Autodesk Fusion 360 part; units mm, degrees
(part 6 of 18)
  arc A594 (213.8474, -42.2017) -> (215.0474, -42.2017) centre (214.4474, -42.2017) ccw
  arc A595 (215.0474, -42.2017) -> (213.8474, -42.2017) centre (214.4474, -42.2017) ccw
  arc A596 (210.3474, -44.4557) -> (211.5474, -44.4557) centre (210.9474, -44.4557) ccw
  arc A597 (211.5474, -44.4557) -> (210.3474, -44.4557) centre (210.9474, -44.4557) ccw
  arc A598 (215.0474, -23.1516) -> (213.8474, -23.1516) centre (214.4474, -23.1516) ccw
  arc A599 (213.8474, -23.1516) -> (215.0474, -23.1516) centre (214.4474, -23.1516) ccw
  arc A600 (211.5474, -25.4057) -> (210.3474, -25.4057) centre (210.9474, -25.4057) ccw
  arc A601 (210.3474, -25.4057) -> (211.5474, -25.4057) centre (210.9474, -25.4057) ccw
  arc A602 (213.8474, -80.3272) -> (215.0474, -80.3272) centre (214.4474, -80.3272) ccw
  arc A603 (215.0474, -80.3272) -> (213.8474, -80.3272) centre (214.4474, -80.3272) ccw
  arc A604 (210.3474, -82.5812) -> (211.5474, -82.5812) centre (210.9474, -82.5812) ccw
  arc A605 (211.5474, -82.5812) -> (210.3474, -82.5812) centre (210.9474, -82.5812) ccw
  arc A606 (195.9974, -42.2017) -> (194.7974, -42.2017) centre (195.3974, -42.2017) ccw
  arc A607 (194.7974, -42.2017) -> (195.9974, -42.2017) centre (195.3974, -42.2017) ccw
  arc A608 (192.4974, -44.4557) -> (191.2974, -44.4557) centre (191.8974, -44.4557) ccw
  arc A609 (191.2974, -44.4557) -> (192.4974, -44.4557) centre (191.8974, -44.4557) ccw
  arc A610 (175.1224, -4.318) -> (176.9224, -4.318) centre (176.0224, -4.318) ccw
  arc A611 (176.9224, -4.318) -> (175.1224, -4.318) centre (176.0224, -4.318) ccw
  line L3563 (172.5823, -3.418) -> (174.3823, -3.418)
  line L3564 (174.3823, -5.218) -> (172.5823, -5.218)
  line L3565 (172.5823, -5.218) -> (172.5823, -3.418)
  line L3566 (174.3823, -3.418) -> (174.3823, -5.218)
  line L3567 (184.8974, -50.5184) -> (198.8974, -50.5184)
  line L3568 (198.8974, -50.5184) -> (198.8974, -64.5184)
  line L3569 (184.8974, -64.5184) -> (184.8974, -50.5184)
  line L3570 (198.8974, -64.5184) -> (184.8974, -64.5184)
  line L3571 (179.8474, -69.5811) -> (179.8474, -83.5812)
  line L3572 (165.8473, -83.5812) -> (165.8473, -69.5811)
  line L3573 (165.8473, -69.5811) -> (179.8474, -69.5811)
  line L3574 (179.8474, -83.5812) -> (165.8473, -83.5812)
  line L3575 (165.8473, -50.5184) -> (179.8474, -50.5184)
  line L3576 (165.8473, -64.5184) -> (165.8473, -50.5184)
  line L3577 (179.8474, -50.5184) -> (179.8474, -64.5184)
  line L3578 (179.8474, -64.5184) -> (165.8473, -64.5184)
  line L3579 (179.8474, -45.4557) -> (165.8473, -45.4557)
  line L3580 (179.8474, -31.4557) -> (179.8474, -45.4557)
  line L3581 (165.8473, -45.4557) -> (165.8473, -31.4557)
  line L3582 (165.8473, -31.4557) -> (179.8474, -31.4557)
  line L3583 (179.8474, -26.4057) -> (165.8473, -26.4057)
  line L3584 (179.8474, -12.4056) -> (179.8474, -26.4057)
  line L3585 (165.8473, -26.4057) -> (165.8473, -12.4056)
  line L3586 (165.8473, -12.4056) -> (179.8474, -12.4056)
  line L3587 (160.7973, -83.5812) -> (146.7973, -83.5812)
  line L3588 (146.7973, -69.5811) -> (160.7973, -69.5811)
  line L3589 (160.7973, -69.5811) -> (160.7973, -83.5812)
  line L3590 (146.7973, -83.5812) -> (146.7973, -69.5811)
  line L3591 (160.7973, -45.4557) -> (146.7973, -45.4557)
  line L3592 (146.7973, -45.4557) -> (146.7973, -31.4557)
  line L3593 (160.7973, -31.4557) -> (160.7973, -45.4557)
  line L3594 (146.7973, -31.4557) -> (160.7973, -31.4557)
  line L3595 (160.7973, -50.5184) -> (160.7973, -64.5184)
  line L3596 (160.7973, -64.5184) -> (146.7973, -64.5184)
  line L3597 (146.7973, -64.5184) -> (146.7973, -50.5184)
  line L3598 (146.7973, -50.5184) -> (160.7973, -50.5184)
  line L3599 (160.7973, -12.4056) -> (160.7973, -26.4057)
  line L3600 (146.7973, -12.4056) -> (160.7973, -12.4056)
  line L3601 (146.7973, -26.4057) -> (146.7973, -12.4056)
  line L3602 (160.7973, -26.4057) -> (146.7973, -26.4057)
  line L3603 (141.7473, -64.5184) -> (127.7473, -64.5184)
  line L3604 (141.7473, -50.5184) -> (141.7473, -64.5184)
  line L3605 (127.7473, -50.5184) -> (141.7473, -50.5184)
  line L3606 (127.7473, -64.5184) -> (127.7473, -50.5184)
  line L3607 (141.7473, -45.4557) -> (127.7473, -45.4557)
  line L3608 (127.7473, -45.4557) -> (127.7473, -31.4557)
  line L3609 (141.7473, -31.4557) -> (141.7473, -45.4557)
  line L3610 (127.7473, -31.4557) -> (141.7473, -31.4557)
  line L3611 (127.7473, -12.4056) -> (141.7473, -12.4056)
  line L3612 (141.7473, -12.4056) -> (141.7473, -26.4057)
  line L3613 (141.7473, -26.4057) -> (127.7473, -26.4057)
  line L3614 (127.7473, -26.4057) -> (127.7473, -12.4056)
  line L3615 (141.7473, -83.5812) -> (127.7473, -83.5812)
  line L3616 (127.7473, -83.5812) -> (127.7473, -69.5811)
  line L3617 (127.7473, -69.5811) -> (141.7473, -69.5811)
  line L3618 (141.7473, -69.5811) -> (141.7473, -83.5812)
  line L3619 (108.6972, -69.5811) -> (122.6972, -69.5811)
  line L3620 (122.6972, -83.5812) -> (108.6972, -83.5812)
  line L3621 (108.6972, -83.5812) -> (108.6972, -69.5811)
  line L3622 (122.6972, -69.5811) -> (122.6972, -83.5812)
  line L3623 (108.6972, -64.5184) -> (108.6972, -50.5184)
  line L3624 (122.6972, -64.5184) -> (108.6972, -64.5184)
  line L3625 (122.6972, -50.5184) -> (122.6972, -64.5184)
  line L3626 (108.6972, -50.5184) -> (122.6972, -50.5184)
  line L3627 (108.6972, -12.4056) -> (122.6972, -12.4056)
  line L3628 (108.6972, -26.4057) -> (108.6972, -12.4056)
  line L3629 (122.6972, -26.4057) -> (108.6972, -26.4057)
  line L3630 (122.6972, -12.4056) -> (122.6972, -26.4057)
  line L3631 (122.6972, -45.4557) -> (108.6972, -45.4557)
  line L3632 (122.6972, -31.4557) -> (122.6972, -45.4557)
  line L3633 (108.6972, -31.4557) -> (122.6972, -31.4557)
  line L3634 (108.6972, -45.4557) -> (108.6972, -31.4557)
  line L3635 (89.6472, -26.4057) -> (89.6472, -12.4056)
  line L3636 (103.6472, -12.4056) -> (103.6472, -26.4057)
  line L3637 (103.6472, -26.4057) -> (89.6472, -26.4057)
  line L3638 (89.6472, -12.4056) -> (103.6472, -12.4056)
  line L3639 (89.6472, -31.4557) -> (103.6472, -31.4557)
  line L3640 (89.6472, -45.4557) -> (89.6472, -31.4557)
  line L3641 (103.6472, -31.4557) -> (103.6472, -45.4557)
  line L3642 (103.6472, -45.4557) -> (89.6472, -45.4557)
  line L3643 (89.6472, -83.5812) -> (89.6472, -69.5811)
  line L3644 (103.6472, -83.5812) -> (89.6472, -83.5812)
  line L3645 (89.6472, -69.5811) -> (103.6472, -69.5811)
  line L3646 (103.6472, -69.5811) -> (103.6472, -83.5812)
  line L3647 (103.6472, -64.5184) -> (89.6472, -64.5184)
  line L3648 (89.6472, -50.5184) -> (103.6472, -50.5184)
  line L3649 (103.6472, -50.5184) -> (103.6472, -64.5184)
  line L3650 (89.6472, -64.5184) -> (89.6472, -50.5184)
  line L3651 (198.8974, -69.5811) -> (198.8974, -83.5812)
  line L3652 (184.8974, -83.5812) -> (184.8974, -69.5811)
  line L3653 (184.8974, -69.5811) -> (198.8974, -69.5811)
  line L3654 (198.8974, -83.5812) -> (184.8974, -83.5812)
  line L3655 (198.8974, -26.4057) -> (184.8974, -26.4057)
  line L3656 (184.8974, -12.4056) -> (198.8974, -12.4056)
  line L3657 (198.8974, -12.4056) -> (198.8974, -26.4057)
  line L3658 (184.8974, -26.4057) -> (184.8974, -12.4056)
  line L3659 (84.5972, -83.5812) -> (70.5971, -83.5812)
  line L3660 (70.5971, -69.5811) -> (84.5972, -69.5811)
  line L3661 (84.5972, -69.5811) -> (84.5972, -83.5812)
  line L3662 (70.5971, -83.5812) -> (70.5971, -69.5811)
  line L3663 (84.5972, -45.4557) -> (70.5971, -45.4557)
  line L3664 (84.5972, -31.4557) -> (84.5972, -45.4557)
  line L3665 (70.5971, -31.4557) -> (84.5972, -31.4557)
  line L3666 (70.5971, -45.4557) -> (70.5971, -31.4557)
  line L3667 (84.5972, -12.4056) -> (84.5972, -26.4057)
  line L3668 (84.5972, -26.4057) -> (70.5971, -26.4057)
  line L3669 (70.5971, -26.4057) -> (70.5971, -12.4056)
  line L3670 (70.5971, -12.4056) -> (84.5972, -12.4056)
  line L3671 (70.5971, -64.5184) -> (70.5971, -50.5184)
  line L3672 (84.5972, -64.5184) -> (70.5971, -64.5184)
  line L3673 (70.5971, -50.5184) -> (84.5972, -50.5184)
  line L3674 (84.5972, -50.5184) -> (84.5972, -64.5184)
  line L3675 (65.5471, -83.5812) -> (51.5471, -83.5812)
  line L3676 (51.5471, -69.5811) -> (65.5471, -69.5811)
  line L3677 (65.5471, -69.5811) -> (65.5471, -83.5812)
  line L3678 (51.5471, -83.5812) -> (51.5471, -69.5811)
  line L3679 (51.5471, -50.5184) -> (65.5471, -50.5184)
  line L3680 (65.5471, -64.5184) -> (51.5471, -64.5184)
  line L3681 (65.5471, -50.5184) -> (65.5471, -64.5184)
  line L3682 (51.5471, -64.5184) -> (51.5471, -50.5184)
  line L3683 (51.5471, -31.4557) -> (65.5471, -31.4557)
  line L3684 (65.5471, -45.4557) -> (51.5471, -45.4557)
  line L3685 (51.5471, -45.4557) -> (51.5471, -31.4557)
  line L3686 (65.5471, -31.4557) -> (65.5471, -45.4557)
  line L3687 (32.4971, -64.5184) -> (32.4971, -50.5184)
  line L3688 (32.4971, -50.5184) -> (46.4971, -50.5184)
  line L3689 (46.4971, -50.5184) -> (46.4971, -64.5184)
  line L3690 (46.4971, -64.5184) -> (32.4971, -64.5184)
  line L3691 (32.4971, -83.5812) -> (32.4971, -69.5811)
  line L3692 (46.4971, -69.5811) -> (46.4971, -83.5812)
  line L3693 (32.4971, -69.5811) -> (46.4971, -69.5811)
  line L3694 (46.4971, -83.5812) -> (32.4971, -83.5812)
  line L3695 (13.447, -83.5812) -> (13.447, -69.5811)
  line L3696 (13.447, -69.5811) -> (27.4471, -69.5811)
  line L3697 (27.4471, -83.5812) -> (13.447, -83.5812)
  line L3698 (27.4471, -69.5811) -> (27.4471, -83.5812)
  line L3699 (-5.603, -83.5812) -> (-5.603, -69.5811)
  line L3700 (8.397, -83.5812) -> (-5.603, -83.5812)
  line L3701 (8.397, -69.5811) -> (8.397, -83.5812)
  line L3702 (-5.603, -69.5811) -> (8.397, -69.5811)
  line L3703 (65.5471, -12.4056) -> (65.5471, -26.4057)
  line L3704 (65.5471, -26.4057) -> (51.5471, -26.4057)
  line L3705 (51.5471, -12.4056) -> (65.5471, -12.4056)
  line L3706 (51.5471, -26.4057) -> (51.5471, -12.4056)
  line L3707 (46.4971, -31.4557) -> (46.4971, -45.4557)
  line L3708 (46.4971, -45.4557) -> (32.4971, -45.4557)
  line L3709 (32.4971, -31.4557) -> (46.4971, -31.4557)
  line L3710 (32.4971, -45.4557) -> (32.4971, -31.4557)
  line L3711 (46.4971, -26.4057) -> (32.4971, -26.4057)
  line L3712 (32.4971, -12.4056) -> (46.4971, -12.4056)
  line L3713 (46.4971, -12.4056) -> (46.4971, -26.4057)
  line L3714 (32.4971, -26.4057) -> (32.4971, -12.4056)
  line L3715 (13.447, -26.4057) -> (13.447, -12.4056)
  line L3716 (13.447, -12.4056) -> (27.4471, -12.4056)
  line L3717 (27.4471, -26.4057) -> (13.447, -26.4057)
  line L3718 (27.4471, -12.4056) -> (27.4471, -26.4057)
  line L3719 (13.447, -64.5184) -> (13.447, -50.5184)
  line L3720 (27.4471, -50.5184) -> (27.4471, -64.5184)
  line L3721 (13.447, -50.5184) -> (27.4471, -50.5184)
  line L3722 (27.4471, -64.5184) -> (13.447, -64.5184)
  line L3723 (13.447, -31.4557) -> (27.4471, -31.4557)
  line L3724 (27.4471, -31.4557) -> (27.4471, -45.4557)
  line L3725 (13.447, -45.4557) -> (13.447, -31.4557)
  line L3726 (27.4471, -45.4557) -> (13.447, -45.4557)
  line L3727 (-5.603, -12.4056) -> (8.397, -12.4056)
  line L3728 (-5.603, -26.4057) -> (-5.603, -12.4056)
  line L3729 (8.397, -12.4056) -> (8.397, -26.4057)
  line L3730 (8.397, -26.4057) -> (-5.603, -26.4057)
  line L3731 (-5.603, -45.4557) -> (-5.603, -31.4557)
  line L3732 (8.397, -31.4557) -> (8.397, -45.4557)
  line L3733 (-5.603, -31.4557) -> (8.397, -31.4557)
  line L3734 (8.397, -45.4557) -> (-5.603, -45.4557)
  line L3735 (-5.603, -50.5184) -> (8.397, -50.5184)
  line L3736 (-5.603, -64.5184) -> (-5.603, -50.5184)
  line L3737 (8.397, -50.5184) -> (8.397, -64.5184)
  line L3738 (8.397, -64.5184) -> (-5.603, -64.5184)
  line L3739 (203.9474, -64.5184) -> (203.9474, -50.5184)
  line L3740 (217.9474, -64.5184) -> (203.9474, -64.5184)
  line L3741 (217.9474, -50.5184) -> (217.9474, -64.5184)
  line L3742 (203.9474, -50.5184) -> (217.9474, -50.5184)
  line L3743 (203.9474, -45.4557) -> (203.9474, -31.4557)
  line L3744 (203.9474, -31.4557) -> (217.9474, -31.4557)
  line L3745 (217.9474, -31.4557) -> (217.9474, -45.4557)
  line L3746 (217.9474, -45.4557) -> (203.9474, -45.4557)
  line L3747 (203.9474, -12.4056) -> (217.9474, -12.4056)
  line L3748 (217.9474, -12.4056) -> (217.9474, -26.4057)
  line L3749 (203.9474, -26.4057) -> (203.9474, -12.4056)
  line L3750 (217.9474, -26.4057) -> (203.9474, -26.4057)
  line L3751 (203.9474, -69.5811) -> (217.9474, -69.5811)
  line L3752 (217.9474, -83.5812) -> (203.9474, -83.5812)
  line L3753 (217.9474, -69.5811) -> (217.9474, -83.5812)
  line L3754 (203.9474, -83.5812) -> (203.9474, -69.5811)
  line L3755 (184.8974, -45.4557) -> (184.8974, -31.4557)
  line L3756 (184.8974, -31.4557) -> (198.8974, -31.4557)
  line L3757 (198.8974, -31.4557) -> (198.8974, -45.4557)
  line L3758 (198.8974, -45.4557) -> (184.8974, -45.4557)
  arc A612 (206.9597, -6.1629) -> (207.1096, -6.1629) centre (207.0347, -6.1629) ccw
  arc A613 (207.1096, -6.1629) -> (206.9597, -6.1629) centre (207.0347, -6.1629) ccw
  arc A614 (212.2667, -3.8099) -> (212.0665, -3.8099) centre (212.1666, -3.8099) ccw
  arc A615 (212.0665, -3.8099) -> (212.2667, -3.8099) centre (212.1666, -3.8099) ccw
  arc A616 (-2.1624, -5.4611) -> (6.4883, -5.4611) centre (2.1629, -5.4611) ccw
  arc A617 (6.4883, -5.4611) -> (-2.1624, -5.4611) centre (2.1629, -5.4611) ccw
  arc A618 (5.5157, -5.4611) -> (-1.1899, -5.4611) centre (2.1629, -5.4611) ccw
  arc A619 (-1.1899, -5.4611) -> (5.5157, -5.4611) centre (2.1629, -5.4611) ccw
  arc A620 (5.2109, -5.4611) -> (-0.8851, -5.4611) centre (2.1629, -5.4611) ccw
  arc A621 (-0.8851, -5.4611) -> (5.2109, -5.4611) centre (2.1629, -5.4611) ccw
  line L3759 (181.2044, -1.3566) -> (181.2044, -3.0235)
  line L3760 (181.2044, 2.4608) -> (181.2044, 0.9765)
  line L3761 (190.1444, -1.3566) -> (190.1444, -3.0235)
  line L3762 (190.1444, 2.411) -> (190.1444, 0.9765)
  line L3763 (181.2044, 2.4608) -> (190.1444, 2.411)
  line L3764 (200.2342, -1.2444) -> (199.2753, -1.2444)
  line L3765 (199.2753, -1.2444) -> (199.2753, -2.5656)
  line L3766 (199.2753, -2.5656) -> (200.2342, -2.5656)
  line L3767 (201.0866, -1.2444) -> (202.0455, -1.2444)
  line L3768 (202.0455, -1.2444) -> (202.0455, -2.5656)
  line L3769 (202.0455, -2.5656) -> (201.0866, -2.5656)
  line L3770 (213.977, -5.1867) -> (214.6507, -5.1867)
  line L3771 (214.6507, -5.1867) -> (214.6507, -5.8604)
  line L3772 (213.977, -12.3392) -> (214.6507, -12.3392)
  line L3773 (214.6507, -12.3392) -> (214.6507, -11.6655)
  line L3774 (208.172, -5.1867) -> (207.4983, -5.1867)
  line L3775 (207.4983, -5.1867) -> (207.4983, -5.8604)
  line L3776 (208.172, -12.3392) -> (207.4983, -12.3392)
  line L3777 (207.4983, -12.3392) -> (207.4983, -11.6655)
  line L3778 (188.1326, -7.3916) -> (189.0915, -7.3916)
  line L3779 (189.0915, -7.3916) -> (189.0915, -6.0704)
  line L3780 (189.0915, -6.0704) -> (188.1326, -6.0704)
  line L3781 (187.2802, -7.3916) -> (186.3213, -7.3916)
  line L3782 (186.3213, -7.3916) -> (186.3213, -6.0704)
  line L3783 (186.3213, -6.0704) -> (187.2802, -6.0704)
  line L3784 (182.7082, -6.0704) -> (181.7493, -6.0704)
  line L3785 (181.7493, -6.0704) -> (181.7493, -7.3916)
  line L3786 (181.7493, -7.3916) -> (182.7082, -7.3916)
  line L3787 (183.5606, -6.0704) -> (184.5195, -6.0704)
  line L3788 (184.5195, -6.0704) -> (184.5195, -7.3916)
  line L3789 (184.5195, -7.3916) -> (183.5606, -7.3916)
  line L3790 (208.6489, -3.8645) -> (208.6489, -0.7644)
  line L3791 (211.749, -0.7644) -> (208.6489, -0.7644)
  line L3792 (211.7477, -3.8645) -> (211.7477, -0.7644)
  line L3793 (208.6489, -3.8886) -> (209.4871, -3.8886)
  line L3794 (210.9095, -3.8886) -> (211.7477, -3.8886)
  arc A622 (209.5125, -3.8886) -> (210.9095, -3.8886) centre (210.211, -4.1061) cw
  line L3795 (141.7615, -77.4607) -> (141.7615, -77.7869)
  line L3796 (141.7615, -75.9344) -> (141.7615, -76.2604)
  line L3797 (138.9091, -75.9344) -> (141.7615, -75.9344)
  line L3798 (138.9091, -77.7869) -> (141.7615, -77.7869)
  line L3799 (139.3639, -77.7867) -> (139.3639, -75.9343)
  line L3800 (138.6805, -77.3568) -> (138.6805, -77.863)
  line L3801 (138.9853, -77.3568) -> (138.6805, -77.3568)
  line L3802 (138.6805, -77.863) -> (138.9853, -77.863)
  line L3803 (138.9853, -77.863) -> (138.9853, -77.3568)
  line L3804 (138.6805, -76.3644) -> (138.6805, -75.8582)
  line L3805 (138.9853, -75.8582) -> (138.9853, -76.3644)
  line L3806 (138.9853, -76.3644) -> (138.6805, -76.3644)
  line L3807 (138.6805, -75.8582) -> (138.9853, -75.8582)
  line L3808 (141.7615, -20.2852) -> (141.7615, -20.6114)
  line L3809 (141.7615, -18.7589) -> (141.7615, -19.0849)
  line L3810 (138.9091, -18.7589) -> (141.7615, -18.7589)
  line L3811 (138.9091, -20.6114) -> (141.7615, -20.6114)
  line L3812 (139.3639, -20.6112) -> (139.3639, -18.7588)
  line L3813 (138.6805, -20.6874) -> (138.9853, -20.6874)
  line L3814 (138.6805, -20.1812) -> (138.6805, -20.6874)
  line L3815 (138.9853, -20.6874) -> (138.9853, -20.1812)
  line L3816 (138.9853, -20.1812) -> (138.6805, -20.1812)
  line L3817 (138.9853, -19.1888) -> (138.6805, -19.1888)
  line L3818 (138.6805, -19.1888) -> (138.6805, -18.6826)
  line L3819 (138.9853, -18.6826) -> (138.9853, -19.1888)
  line L3820 (138.6805, -18.6826) -> (138.9853, -18.6826)
  line L3821 (141.7615, -39.3352) -> (141.7615, -39.6614)
  line L3822 (141.7615, -37.8089) -> (141.7615, -38.135)
  line L3823 (138.9091, -37.8089) -> (141.7615, -37.8089)
  line L3824 (138.9091, -39.6614) -> (141.7615, -39.6614)
  line L3825 (139.3639, -39.6613) -> (139.3639, -37.8089)
  line L3826 (138.9853, -39.7375) -> (138.9853, -39.2313)
  line L3827 (138.6805, -39.7375) -> (138.9853, -39.7375)
  line L3828 (138.9853, -39.2313) -> (138.6805, -39.2313)
  line L3829 (138.6805, -39.2313) -> (138.6805, -39.7375)
  line L3830 (138.6805, -37.7327) -> (138.9853, -37.7327)
  line L3831 (138.9853, -38.2389) -> (138.6805, -38.2389)
  line L3832 (138.6805, -38.2389) -> (138.6805, -37.7327)
  line L3833 (138.9853, -37.7327) -> (138.9853, -38.2389)
  line L3834 (141.7615, -58.3979) -> (141.7615, -58.7242)
  line L3835 (141.7615, -56.8716) -> (141.7615, -57.1977)
  line L3836 (138.9091, -56.8716) -> (141.7615, -56.8716)
  line L3837 (138.9091, -58.7242) -> (141.7615, -58.7242)
  line L3838 (139.3639, -58.724) -> (139.3639, -56.8716)
  line L3839 (138.6805, -58.8002) -> (138.9853, -58.8002)
  line L3840 (138.9853, -58.8002) -> (138.9853, -58.294)
  line L3841 (138.9853, -58.294) -> (138.6805, -58.294)
  line L3842 (138.6805, -58.294) -> (138.6805, -58.8002)
  line L3843 (138.6805, -56.7954) -> (138.9853, -56.7954)
  line L3844 (138.9853, -57.3016) -> (138.6805, -57.3016)
  line L3845 (138.6805, -57.3016) -> (138.6805, -56.7954)
  line L3846 (138.9853, -56.7954) -> (138.9853, -57.3016)
  line L3847 (160.8115, -20.2852) -> (160.8115, -20.6114)
  line L3848 (160.8115, -18.7589) -> (160.8115, -19.0849)
  line L3849 (157.9591, -18.7589) -> (160.8115, -18.7589)
  line L3850 (157.9591, -20.6114) -> (160.8115, -20.6114)
  line L3851 (158.4139, -20.6112) -> (158.4139, -18.7588)
  line L3852 (158.0353, -20.1812) -> (157.7305, -20.1812)
  line L3853 (157.7305, -20.1812) -> (157.7305, -20.6874)
  line L3854 (157.7305, -20.6874) -> (158.0353, -20.6874)
  line L3855 (158.0353, -20.6874) -> (158.0353, -20.1812)
  line L3856 (157.7305, -18.6826) -> (158.0353, -18.6826)
  line L3857 (157.7305, -19.1888) -> (157.7305, -18.6826)
  line L3858 (158.0353, -19.1888) -> (157.7305, -19.1888)
  line L3859 (158.0353, -18.6826) -> (158.0353, -19.1888)
  line L3860 (160.8115, -77.4607) -> (160.8115, -77.7869)
  line L3861 (160.8115, -75.9344) -> (160.8115, -76.2604)
  line L3862 (157.9591, -75.9344) -> (160.8115, -75.9344)
  line L3863 (157.9591, -77.7869) -> (160.8115, -77.7869)
  line L3864 (158.4139, -77.7867) -> (158.4139, -75.9343)
  line L3865 (157.7305, -77.863) -> (158.0353, -77.863)
  line L3866 (158.0353, -77.863) -> (158.0353, -77.3568)
  line L3867 (158.0353, -77.3568) -> (157.7305, -77.3568)
  line L3868 (157.7305, -77.3568) -> (157.7305, -77.863)
  line L3869 (158.0353, -76.3644) -> (157.7305, -76.3644)
  line L3870 (157.7305, -75.8582) -> (158.0353, -75.8582)
  line L3871 (157.7305, -76.3644) -> (157.7305, -75.8582)
  line L3872 (158.0353, -75.8582) -> (158.0353, -76.3644)
  line L3873 (160.8115, -58.3979) -> (160.8115, -58.7242)
  line L3874 (160.8115, -56.8716) -> (160.8115, -57.1977)
  line L3875 (157.9591, -56.8716) -> (160.8115, -56.8716)
  line L3876 (157.9591, -58.7242) -> (160.8115, -58.7242)
  line L3877 (158.4139, -58.724) -> (158.4139, -56.8716)
  line L3878 (158.0353, -58.8002) -> (158.0353, -58.294)
  line L3879 (158.0353, -58.294) -> (157.7305, -58.294)
  line L3880 (157.7305, -58.8002) -> (158.0353, -58.8002)
  line L3881 (157.7305, -58.294) -> (157.7305, -58.8002)
  line L3882 (158.0353, -56.7954) -> (158.0353, -57.3016)
  line L3883 (157.7305, -56.7954) -> (158.0353, -56.7954)
  line L3884 (157.7305, -57.3016) -> (157.7305, -56.7954)
  line L3885 (158.0353, -57.3016) -> (157.7305, -57.3016)
  line L3886 (160.8115, -39.3352) -> (160.8115, -39.6614)
  line L3887 (160.8115, -37.8089) -> (160.8115, -38.135)
  line L3888 (157.9591, -37.8089) -> (160.8115, -37.8089)
  line L3889 (157.9591, -39.6614) -> (160.8115, -39.6614)
  line L3890 (158.4139, -39.6613) -> (158.4139, -37.8089)
  line L3891 (158.0353, -39.2313) -> (157.7305, -39.2313)
  line L3892 (157.7305, -39.2313) -> (157.7305, -39.7375)
  line L3893 (158.0353, -39.7375) -> (158.0353, -39.2313)
  line L3894 (157.7305, -39.7375) -> (158.0353, -39.7375)
  line L3895 (158.0353, -37.7327) -> (158.0353, -38.2389)
  line L3896 (157.7305, -37.7327) -> (158.0353, -37.7327)
  line L3897 (158.0353, -38.2389) -> (157.7305, -38.2389)
  line L3898 (157.7305, -38.2389) -> (157.7305, -37.7327)
  line L3899 (179.8616, -20.2852) -> (179.8616, -20.6114)
  line L3900 (179.8616, -18.7589) -> (179.8616, -19.0849)
  line L3901 (177.0092, -18.7589) -> (179.8616, -18.7589)
  line L3902 (177.0091, -20.6114) -> (179.8616, -20.6114)
  line L3903 (177.464, -20.6112) -> (177.464, -18.7588)
  line L3904 (177.0854, -20.1812) -> (176.7806, -20.1812)
  line L3905 (177.0854, -20.6874) -> (177.0854, -20.1812)
  line L3906 (176.7806, -20.6874) -> (177.0854, -20.6874)
  line L3907 (176.7806, -20.1812) -> (176.7806, -20.6874)
  line L3908 (177.0854, -19.1888) -> (176.7806, -19.1888)
  line L3909 (176.7806, -19.1888) -> (176.7806, -18.6826)
  line L3910 (176.7806, -18.6826) -> (177.0854, -18.6826)
  line L3911 (177.0854, -18.6826) -> (177.0854, -19.1888)
  line L3912 (179.8616, -77.4607) -> (179.8616, -77.7869)
  line L3913 (179.8616, -75.9344) -> (179.8616, -76.2604)
  line L3914 (177.0092, -75.9344) -> (179.8616, -75.9344)
  line L3915 (177.0091, -77.7869) -> (179.8616, -77.7869)
  line L3916 (177.464, -77.7867) -> (177.464, -75.9343)
  line L3917 (176.7806, -77.3568) -> (176.7806, -77.863)
  line L3918 (177.0854, -77.3568) -> (176.7806, -77.3568)
  line L3919 (176.7806, -77.863) -> (177.0854, -77.863)
  line L3920 (177.0854, -77.863) -> (177.0854, -77.3568)
  line L3921 (176.7806, -76.3644) -> (176.7806, -75.8582)
  line L3922 (177.0854, -75.8582) -> (177.0854, -76.3644)
  line L3923 (176.7806, -75.8582) -> (177.0854, -75.8582)
  line L3924 (177.0854, -76.3644) -> (176.7806, -76.3644)
  line L3925 (179.8616, -58.3979) -> (179.8616, -58.7242)
  line L3926 (179.8616, -56.8716) -> (179.8616, -57.1977)
  line L3927 (177.0092, -56.8716) -> (179.8616, -56.8716)
  line L3928 (177.0091, -58.7242) -> (179.8616, -58.7242)
  line L3929 (177.464, -58.724) -> (177.464, -56.8716)
  line L3930 (177.0854, -58.294) -> (176.7806, -58.294)
  line L3931 (176.7806, -58.8002) -> (177.0854, -58.8002)
  line L3932 (177.0854, -58.8002) -> (177.0854, -58.294)
  line L3933 (176.7806, -58.294) -> (176.7806, -58.8002)
  line L3934 (177.0854, -56.7954) -> (177.0854, -57.3016)
  line L3935 (177.0854, -57.3016) -> (176.7806, -57.3016)
  line L3936 (176.7806, -57.3016) -> (176.7806, -56.7954)
  line L3937 (176.7806, -56.7954) -> (177.0854, -56.7954)
  line L3938 (179.8616, -39.3352) -> (179.8616, -39.6614)
  line L3939 (179.8616, -37.8089) -> (179.8616, -38.135)
  line L3940 (177.0092, -37.8089) -> (179.8616, -37.8089)
  line L3941 (177.0091, -39.6614) -> (179.8616, -39.6614)
  line L3942 (177.464, -39.6613) -> (177.464, -37.8089)
  line L3943 (176.7806, -39.7375) -> (177.0854, -39.7375)
  line L3944 (177.0854, -39.7375) -> (177.0854, -39.2313)
  line L3945 (176.7806, -39.2313) -> (176.7806, -39.7375)
  line L3946 (177.0854, -39.2313) -> (176.7806, -39.2313)
  line L3947 (176.7806, -37.7327) -> (177.0854, -37.7327)
  line L3948 (176.7806, -38.2389) -> (176.7806, -37.7327)
  line L3949 (177.0854, -37.7327) -> (177.0854, -38.2389)
  line L3950 (177.0854, -38.2389) -> (176.7806, -38.2389)
  line L3951 (103.6614, -77.4607) -> (103.6614, -77.7869)
  line L3952 (103.6614, -75.9344) -> (103.6614, -76.2604)
  line L3953 (100.809, -75.9344) -> (103.6614, -75.9344)
  line L3954 (100.809, -77.7869) -> (103.6614, -77.7869)
  line L3955 (101.2638, -77.7867) -> (101.2638, -75.9343)
  line L3956 (100.5804, -77.863) -> (100.8852, -77.863)
  line L3957 (100.8852, -77.3568) -> (100.5804, -77.3568)
  line L3958 (100.8852, -77.863) -> (100.8852, -77.3568)
  line L3959 (100.5804, -77.3568) -> (100.5804, -77.863)
  line L3960 (100.8852, -76.3644) -> (100.5804, -76.3644)
  line L3961 (100.8852, -75.8582) -> (100.8852, -76.3644)
  line L3962 (100.5804, -76.3644) -> (100.5804, -75.8582)
  line L3963 (100.5804, -75.8582) -> (100.8852, -75.8582)
  line L3964 (103.6614, -58.3979) -> (103.6614, -58.7242)
  line L3965 (103.6614, -56.8716) -> (103.6614, -57.1977)
  line L3966 (100.809, -56.8716) -> (103.6614, -56.8716)
  line L3967 (100.809, -58.7242) -> (103.6614, -58.7242)
  line L3968 (101.2638, -58.724) -> (101.2638, -56.8716)
  line L3969 (100.8852, -58.8002) -> (100.8852, -58.294)
  line L3970 (100.8852, -58.294) -> (100.5804, -58.294)
  line L3971 (100.5804, -58.8002) -> (100.8852, -58.8002)
  line L3972 (100.5804, -58.294) -> (100.5804, -58.8002)
  line L3973 (100.5804, -56.7954) -> (100.8852, -56.7954)
  line L3974 (100.5804, -57.3016) -> (100.5804, -56.7954)
  line L3975 (100.8852, -56.7954) -> (100.8852, -57.3016)
  line L3976 (100.8852, -57.3016) -> (100.5804, -57.3016)
  line L3977 (103.6614, -20.2852) -> (103.6614, -20.6114)
  line L3978 (103.6614, -18.7589) -> (103.6614, -19.0849)
  line L3979 (100.809, -18.7589) -> (103.6614, -18.7589)
  line L3980 (100.809, -20.6114) -> (103.6614, -20.6114)
  line L3981 (101.2638, -20.6112) -> (101.2638, -18.7588)
  line L3982 (100.8852, -20.1812) -> (100.5804, -20.1812)
  line L3983 (100.8852, -20.6874) -> (100.8852, -20.1812)
  line L3984 (100.5804, -20.6874) -> (100.8852, -20.6874)
  line L3985 (100.5804, -20.1812) -> (100.5804, -20.6874)
  line L3986 (100.8852, -18.6826) -> (100.8852, -19.1888)
  line L3987 (100.5804, -19.1888) -> (100.5804, -18.6826)
  line L3988 (100.5804, -18.6826) -> (100.8852, -18.6826)
  line L3989 (100.8852, -19.1888) -> (100.5804, -19.1888)
  line L3990 (103.6614, -39.3352) -> (103.6614, -39.6614)
  line L3991 (103.6614, -37.8089) -> (103.6614, -38.135)
  line L3992 (100.809, -37.8089) -> (103.6614, -37.8089)
  line L3993 (100.809, -39.6614) -> (103.6614, -39.6614)
  line L3994 (101.2638, -39.6613) -> (101.2638, -37.8089)
  line L3995 (100.5804, -39.7375) -> (100.8852, -39.7375)
  line L3996 (100.5804, -39.2313) -> (100.5804, -39.7375)
  line L3997 (100.8852, -39.7375) -> (100.8852, -39.2313)
  line L3998 (100.8852, -39.2313) -> (100.5804, -39.2313)
  line L3999 (100.5804, -38.2389) -> (100.5804, -37.7327)
  line L4000 (100.8852, -38.2389) -> (100.5804, -38.2389)
  line L4001 (100.8852, -37.7327) -> (100.8852, -38.2389)
  line L4002 (100.5804, -37.7327) -> (100.8852, -37.7327)
  line L4003 (122.7115, -20.2852) -> (122.7115, -20.6114)
  line L4004 (122.7115, -18.7589) -> (122.7115, -19.0849)
  line L4005 (119.8591, -18.7589) -> (122.7115, -18.7589)
  line L4006 (119.859, -20.6114) -> (122.7115, -20.6114)
  line L4007 (120.3138, -20.6112) -> (120.3138, -18.7588)
  line L4008 (119.9352, -20.6874) -> (119.9352, -20.1812)
  line L4009 (119.9352, -20.1812) -> (119.6304, -20.1812)
  line L4010 (119.6304, -20.1812) -> (119.6304, -20.6874)
  line L4011 (119.6304, -20.6874) -> (119.9352, -20.6874)
  line L4012 (119.6304, -18.6826) -> (119.9352, -18.6826)
  line L4013 (119.9352, -19.1888) -> (119.6304, -19.1888)
  line L4014 (119.6304, -19.1888) -> (119.6304, -18.6826)
  line L4015 (119.9352, -18.6826) -> (119.9352, -19.1888)
  line L4016 (122.7115, -58.3979) -> (122.7115, -58.7242)
  line L4017 (122.7115, -56.8716) -> (122.7115, -57.1977)
  line L4018 (119.8591, -56.8716) -> (122.7115, -56.8716)
  line L4019 (119.859, -58.7242) -> (122.7115, -58.7242)
  line L4020 (120.3138, -58.724) -> (120.3138, -56.8716)
  line L4021 (119.6304, -58.294) -> (119.6304, -58.8002)
  line L4022 (119.9352, -58.294) -> (119.6304, -58.294)
  line L4023 (119.6304, -58.8002) -> (119.9352, -58.8002)
  line L4024 (119.9352, -58.8002) -> (119.9352, -58.294)
  line L4025 (119.6304, -57.3016) -> (119.6304, -56.7954)
  line L4026 (119.9352, -56.7954) -> (119.9352, -57.3016)
  line L4027 (119.9352, -57.3016) -> (119.6304, -57.3016)
  line L4028 (119.6304, -56.7954) -> (119.9352, -56.7954)
  line L4029 (122.7115, -39.3352) -> (122.7115, -39.6614)
  line L4030 (122.7115, -37.8089) -> (122.7115, -38.135)
  line L4031 (119.8591, -37.8089) -> (122.7115, -37.8089)
  line L4032 (119.859, -39.6614) -> (122.7115, -39.6614)
  line L4033 (120.3138, -39.6613) -> (120.3138, -37.8089)
  line L4034 (119.6304, -39.7375) -> (119.9352, -39.7375)
  line L4035 (119.9352, -39.7375) -> (119.9352, -39.2313)
  line L4036 (119.6304, -39.2313) -> (119.6304, -39.7375)
  line L4037 (119.9352, -39.2313) -> (119.6304, -39.2313)
  line L4038 (119.9352, -38.2389) -> (119.6304, -38.2389)
  line L4039 (119.9352, -37.7327) -> (119.9352, -38.2389)
  line L4040 (119.6304, -37.7327) -> (119.9352, -37.7327)
  line L4041 (119.6304, -38.2389) -> (119.6304, -37.7327)
  line L4042 (122.7115, -77.4607) -> (122.7115, -77.7869)
  line L4043 (122.7115, -75.9344) -> (122.7115, -76.2604)
  line L4044 (119.8591, -75.9344) -> (122.7115, -75.9344)
  line L4045 (119.859, -77.7869) -> (122.7115, -77.7869)
  line L4046 (120.3138, -77.7867) -> (120.3138, -75.9343)
  line L4047 (119.6304, -77.3568) -> (119.6304, -77.863)
  line L4048 (119.9352, -77.863) -> (119.9352, -77.3568)
  line L4049 (119.6304, -77.863) -> (119.9352, -77.863)
  line L4050 (119.9352, -77.3568) -> (119.6304, -77.3568)
  line L4051 (119.9352, -75.8582) -> (119.9352, -76.3644)
  line L4052 (119.9352, -76.3644) -> (119.6304, -76.3644)
  line L4053 (119.6304, -75.8582) -> (119.9352, -75.8582)
  line L4054 (119.6304, -76.3644) -> (119.6304, -75.8582)
  line L4055 (8.4112, -77.4607) -> (8.4112, -77.7869)
  line L4056 (8.4112, -75.9344) -> (8.4112, -76.2604)
  line L4057 (5.5588, -75.9344) -> (8.4112, -75.9344)
  line L4058 (5.5588, -77.7869) -> (8.4112, -77.7869)
  line L4059 (6.0136, -77.7867) -> (6.0136, -75.9343)
  line L4060 (5.3302, -77.863) -> (5.635, -77.863)
  line L4061 (5.3302, -77.3568) -> (5.3302, -77.863)
  line L4062 (5.635, -77.863) -> (5.635, -77.3568)
  line L4063 (5.635, -77.3568) -> (5.3302, -77.3568)
  line L4064 (5.3302, -76.3644) -> (5.3302, -75.8582)
  line L4065 (5.3302, -75.8582) -> (5.635, -75.8582)
  line L4066 (5.635, -76.3644) -> (5.3302, -76.3644)
  line L4067 (5.635, -75.8582) -> (5.635, -76.3644)
  line L4068 (27.4613, -77.4607) -> (27.4613, -77.7869)
  line L4069 (27.4613, -75.9344) -> (27.4613, -76.2604)
  line L4070 (24.6089, -75.9344) -> (27.4613, -75.9344)
  line L4071 (24.6088, -77.7869) -> (27.4613, -77.7869)
  line L4072 (25.0637, -77.7867) -> (25.0637, -75.9343)
  line L4073 (24.3803, -77.863) -> (24.6851, -77.863)
  line L4074 (24.3803, -77.3568) -> (24.3803, -77.863)
  line L4075 (24.6851, -77.3568) -> (24.3803, -77.3568)
  line L4076 (24.6851, -77.863) -> (24.6851, -77.3568)
  line L4077 (24.3803, -76.3644) -> (24.3803, -75.8582)
  line L4078 (24.3803, -75.8582) -> (24.6851, -75.8582)
  line L4079 (24.6851, -75.8582) -> (24.6851, -76.3644)
  line L4080 (24.6851, -76.3644) -> (24.3803, -76.3644)
  line L4081 (46.5113, -77.4607) -> (46.5113, -77.7869)
  line L4082 (46.5113, -75.9344) -> (46.5113, -76.2604)
  line L4083 (43.6589, -75.9344) -> (46.5113, -75.9344)
  line L4084 (43.6589, -77.7869) -> (46.5113, -77.7869)
  line L4085 (44.1137, -77.7867) -> (44.1137, -75.9343)
  line L4086 (43.7351, -77.3568) -> (43.4303, -77.3568)
  line L4087 (43.4303, -77.3568) -> (43.4303, -77.863)
  line L4088 (43.4303, -77.863) -> (43.7351, -77.863)
  line L4089 (43.7351, -77.863) -> (43.7351, -77.3568)
  line L4090 (43.7351, -76.3644) -> (43.4303, -76.3644)
  line L4091 (43.4303, -75.8582) -> (43.7351, -75.8582)
  line L4092 (43.7351, -75.8582) -> (43.7351, -76.3644)
  line L4093 (43.4303, -76.3644) -> (43.4303, -75.8582)
  line L4094 (65.5613, -20.2852) -> (65.5613, -20.6114)
  line L4095 (65.5613, -18.7589) -> (65.5613, -19.0849)
  line L4096 (62.7089, -18.7589) -> (65.5613, -18.7589)
  line L4097 (62.7089, -20.6114) -> (65.5613, -20.6114)
  line L4098 (63.1637, -20.6112) -> (63.1637, -18.7588)
  line L4099 (62.7851, -20.6874) -> (62.7851, -20.1812)
  line L4100 (62.7851, -20.1812) -> (62.4803, -20.1812)
  line L4101 (62.4803, -20.6874) -> (62.7851, -20.6874)
  line L4102 (62.4803, -20.1812) -> (62.4803, -20.6874)
  line L4103 (62.4803, -18.6826) -> (62.7851, -18.6826)
  line L4104 (62.4803, -19.1888) -> (62.4803, -18.6826)
  line L4105 (62.7851, -19.1888) -> (62.4803, -19.1888)
  line L4106 (62.7851, -18.6826) -> (62.7851, -19.1888)
  line L4107 (65.5613, -77.4607) -> (65.5613, -77.7869)
  line L4108 (65.5613, -75.9344) -> (65.5613, -76.2604)
  line L4109 (62.7089, -75.9344) -> (65.5613, -75.9344)
  line L4110 (62.7089, -77.7869) -> (65.5613, -77.7869)
  line L4111 (63.1637, -77.7867) -> (63.1637, -75.9343)
  line L4112 (62.7851, -77.863) -> (62.7851, -77.3568)
  line L4113 (62.4803, -77.863) -> (62.7851, -77.863)
  line L4114 (62.7851, -77.3568) -> (62.4803, -77.3568)
  line L4115 (62.4803, -77.3568) -> (62.4803, -77.863)
  line L4116 (62.7851, -75.8582) -> (62.7851, -76.3644)
  line L4117 (62.4803, -76.3644) -> (62.4803, -75.8582)
  line L4118 (62.7851, -76.3644) -> (62.4803, -76.3644)
  line L4119 (62.4803, -75.8582) -> (62.7851, -75.8582)
  line L4120 (65.5613, -39.3352) -> (65.5613, -39.6614)
  line L4121 (65.5613, -37.8089) -> (65.5613, -38.135)
  line L4122 (62.7089, -37.8089) -> (65.5613, -37.8089)
  line L4123 (62.7089, -39.6614) -> (65.5613, -39.6614)
  line L4124 (63.1637, -39.6613) -> (63.1637, -37.8089)
  line L4125 (62.4803, -39.2313) -> (62.4803, -39.7375)
  line L4126 (62.4803, -39.7375) -> (62.7851, -39.7375)
  line L4127 (62.7851, -39.2313) -> (62.4803, -39.2313)
  line L4128 (62.7851, -39.7375) -> (62.7851, -39.2313)
  line L4129 (62.4803, -38.2389) -> (62.4803, -37.7327)
  line L4130 (62.7851, -37.7327) -> (62.7851, -38.2389)
  line L4131 (62.7851, -38.2389) -> (62.4803, -38.2389)
  line L4132 (62.4803, -37.7327) -> (62.7851, -37.7327)
  line L4133 (65.5613, -58.3979) -> (65.5613, -58.7242)
  line L4134 (65.5613, -56.8716) -> (65.5613, -57.1977)
  line L4135 (62.7089, -56.8716) -> (65.5613, -56.8716)
  line L4136 (62.7089, -58.7242) -> (65.5613, -58.7242)
  line L4137 (63.1637, -58.724) -> (63.1637, -56.8716)
  line L4138 (62.4803, -58.8002) -> (62.7851, -58.8002)
  line L4139 (62.7851, -58.8002) -> (62.7851, -58.294)
  line L4140 (62.7851, -58.294) -> (62.4803, -58.294)
  line L4141 (62.4803, -58.294) -> (62.4803, -58.8002)
  line L4142 (62.4803, -56.7954) -> (62.7851, -56.7954)
  line L4143 (62.4803, -57.3016) -> (62.4803, -56.7954)
  line L4144 (62.7851, -56.7954) -> (62.7851, -57.3016)
  line L4145 (62.7851, -57.3016) -> (62.4803, -57.3016)
  line L4146 (84.6114, -39.3352) -> (84.6114, -39.6614)
  line L4147 (84.6114, -37.8089) -> (84.6114, -38.135)
  line L4148 (81.759, -37.8089) -> (84.6114, -37.8089)
  line L4149 (81.759, -39.6614) -> (84.6114, -39.6614)
  line L4150 (82.2138, -39.6613) -> (82.2138, -37.8089)
  line L4151 (81.5304, -39.7375) -> (81.8352, -39.7375)
  line L4152 (81.8352, -39.7375) -> (81.8352, -39.2313)
  line L4153 (81.8352, -39.2313) -> (81.5304, -39.2313)
  line L4154 (81.5304, -39.2313) -> (81.5304, -39.7375)
  line L4155 (81.8352, -38.2389) -> (81.5304, -38.2389)
  line L4156 (81.8352, -37.7327) -> (81.8352, -38.2389)
  line L4157 (81.5304, -37.7327) -> (81.8352, -37.7327)
  line L4158 (81.5304, -38.2389) -> (81.5304, -37.7327)
  line L4159 (84.6114, -77.4607) -> (84.6114, -77.7869)
  line L4160 (84.6114, -75.9344) -> (84.6114, -76.2604)
  line L4161 (81.759, -75.9344) -> (84.6114, -75.9344)
  line L4162 (81.759, -77.7869) -> (84.6114, -77.7869)
  line L4163 (82.2138, -77.7867) -> (82.2138, -75.9343)
  line L4164 (81.5304, -77.3568) -> (81.5304, -77.863)
  line L4165 (81.8352, -77.863) -> (81.8352, -77.3568)
  line L4166 (81.8352, -77.3568) -> (81.5304, -77.3568)
  line L4167 (81.5304, -77.863) -> (81.8352, -77.863)
  line L4168 (81.5304, -75.8582) -> (81.8352, -75.8582)
  line L4169 (81.8352, -75.8582) -> (81.8352, -76.3644)
  line L4170 (81.8352, -76.3644) -> (81.5304, -76.3644)
  line L4171 (81.5304, -76.3644) -> (81.5304, -75.8582)
  line L4172 (84.6114, -20.2852) -> (84.6114, -20.6114)
  line L4173 (84.6114, -18.7589) -> (84.6114, -19.0849)
  line L4174 (81.759, -18.7589) -> (84.6114, -18.7589)
  line L4175 (81.759, -20.6114) -> (84.6114, -20.6114)
  line L4176 (82.2138, -20.6112) -> (82.2138, -18.7588)
  line L4177 (81.8352, -20.1812) -> (81.5304, -20.1812)
  line L4178 (81.5304, -20.1812) -> (81.5304, -20.6874)
  line L4179 (81.8352, -20.6874) -> (81.8352, -20.1812)
  line L4180 (81.5304, -20.6874) -> (81.8352, -20.6874)
  line L4181 (81.5304, -18.6826) -> (81.8352, -18.6826)
  line L4182 (81.5304, -19.1888) -> (81.5304, -18.6826)
  line L4183 (81.8352, -18.6826) -> (81.8352, -19.1888)
  line L4184 (81.8352, -19.1888) -> (81.5304, -19.1888)
  line L4185 (84.6114, -58.3979) -> (84.6114, -58.7242)
  line L4186 (84.6114, -56.8716) -> (84.6114, -57.1977)
  line L4187 (81.759, -56.8716) -> (84.6114, -56.8716)
  line L4188 (81.759, -58.7242) -> (84.6114, -58.7242)
  line L4189 (82.2138, -58.724) -> (82.2138, -56.8716)
  line L4190 (81.8352, -58.8002) -> (81.8352, -58.294)
  line L4191 (81.8352, -58.294) -> (81.5304, -58.294)
  line L4192 (81.5304, -58.294) -> (81.5304, -58.8002)
  line L4193 (81.5304, -58.8002) -> (81.8352, -58.8002)
  line L4194 (81.5304, -57.3016) -> (81.5304, -56.7954)
  line L4195 (81.8352, -57.3016) -> (81.5304, -57.3016)
  line L4196 (81.8352, -56.7954) -> (81.8352, -57.3016)
  line L4197 (81.5304, -56.7954) -> (81.8352, -56.7954)
  line L4198 (8.4112, -58.3979) -> (8.4112, -58.7242)
  line L4199 (8.4112, -56.8716) -> (8.4112, -57.1977)
  line L4200 (5.5588, -56.8716) -> (8.4112, -56.8716)
  line L4201 (5.5588, -58.7242) -> (8.4112, -58.7242)
  line L4202 (6.0136, -58.724) -> (6.0136, -56.8716)
  line L4203 (5.635, -58.8002) -> (5.635, -58.294)
  line L4204 (5.3302, -58.294) -> (5.3302, -58.8002)
  line L4205 (5.635, -58.294) -> (5.3302, -58.294)
  line L4206 (5.3302, -58.8002) -> (5.635, -58.8002)
  line L4207 (5.635, -56.7954) -> (5.635, -57.3016)
  line L4208 (5.635, -57.3016) -> (5.3302, -57.3016)
  line L4209 (5.3302, -57.3016) -> (5.3302, -56.7954)
  line L4210 (5.3302, -56.7954) -> (5.635, -56.7954)
  line L4211 (8.4112, -20.2852) -> (8.4112, -20.6114)
  line L4212 (8.4112, -18.7589) -> (8.4112, -19.0849)
  line L4213 (5.5588, -18.7589) -> (8.4112, -18.7589)
  line L4214 (5.5588, -20.6114) -> (8.4112, -20.6114)
  line L4215 (6.0136, -20.6112) -> (6.0136, -18.7588)
  line L4216 (5.3302, -20.6874) -> (5.635, -20.6874)
  line L4217 (5.3302, -20.1812) -> (5.3302, -20.6874)
  line L4218 (5.635, -20.6874) -> (5.635, -20.1812)
  line L4219 (5.635, -20.1812) -> (5.3302, -20.1812)
  line L4220 (5.3302, -19.1888) -> (5.3302, -18.6826)
  line L4221 (5.635, -19.1888) -> (5.3302, -19.1888)
  line L4222 (5.635, -18.6826) -> (5.635, -19.1888)
  line L4223 (5.3302, -18.6826) -> (5.635, -18.6826)
  line L4224 (8.4112, -39.3352) -> (8.4112, -39.6614)
  line L4225 (8.4112, -37.8089) -> (8.4112, -38.135)
  line L4226 (5.5588, -37.8089) -> (8.4112, -37.8089)
  line L4227 (5.5588, -39.6614) -> (8.4112, -39.6614)
  line L4228 (6.0136, -39.6613) -> (6.0136, -37.8089)
  line L4229 (5.635, -39.2313) -> (5.3302, -39.2313)
  line L4230 (5.3302, -39.7375) -> (5.635, -39.7375)
  line L4231 (5.3302, -39.2313) -> (5.3302, -39.7375)
  line L4232 (5.635, -39.7375) -> (5.635, -39.2313)
  line L4233 (5.635, -38.2389) -> (5.3302, -38.2389)
  line L4234 (5.3302, -38.2389) -> (5.3302, -37.7327)
  line L4235 (5.3302, -37.7327) -> (5.635, -37.7327)
  line L4236 (5.635, -37.7327) -> (5.635, -38.2389)
  line L4237 (27.4613, -39.3352) -> (27.4613, -39.6614)
  line L4238 (27.4613, -37.8089) -> (27.4613, -38.135)
  line L4239 (24.6089, -37.8089) -> (27.4613, -37.8089)
  line L4240 (24.6088, -39.6614) -> (27.4613, -39.6614)
  line L4241 (25.0637, -39.6613) -> (25.0637, -37.8089)
  line L4242 (24.3803, -39.2313) -> (24.3803, -39.7375)
  line L4243 (24.3803, -39.7375) -> (24.6851, -39.7375)
  line L4244 (24.6851, -39.7375) -> (24.6851, -39.2313)
  line L4245 (24.6851, -39.2313) -> (24.3803, -39.2313)
  line L4246 (24.3803, -38.2389) -> (24.3803, -37.7327)
  line L4247 (24.6851, -38.2389) -> (24.3803, -38.2389)
  line L4248 (24.6851, -37.7327) -> (24.6851, -38.2389)
  line L4249 (24.3803, -37.7327) -> (24.6851, -37.7327)
  line L4250 (27.4613, -20.2852) -> (27.4613, -20.6114)
  line L4251 (27.4613, -18.7589) -> (27.4613, -19.0849)
  line L4252 (24.6089, -18.7589) -> (27.4613, -18.7589)
  line L4253 (24.6088, -20.6114) -> (27.4613, -20.6114)
  line L4254 (25.0637, -20.6112) -> (25.0637, -18.7588)
  line L4255 (24.6851, -20.6874) -> (24.6851, -20.1812)
  line L4256 (24.6851, -20.1812) -> (24.3803, -20.1812)
  line L4257 (24.3803, -20.1812) -> (24.3803, -20.6874)
  line L4258 (24.3803, -20.6874) -> (24.6851, -20.6874)
  line L4259 (24.3803, -19.1888) -> (24.3803, -18.6826)
  line L4260 (24.3803, -18.6826) -> (24.6851, -18.6826)
  line L4261 (24.6851, -19.1888) -> (24.3803, -19.1888)
  line L4262 (24.6851, -18.6826) -> (24.6851, -19.1888)
  line L4263 (27.4613, -58.3979) -> (27.4613, -58.7242)
  line L4264 (27.4613, -56.8716) -> (27.4613, -57.1977)
  line L4265 (24.6089, -56.8716) -> (27.4613, -56.8716)
  line L4266 (24.6088, -58.7242) -> (27.4613, -58.7242)
  line L4267 (25.0637, -58.724) -> (25.0637, -56.8716)
  line L4268 (24.6851, -58.294) -> (24.3803, -58.294)
  line L4269 (24.3803, -58.294) -> (24.3803, -58.8002)
  line L4270 (24.3803, -58.8002) -> (24.6851, -58.8002)
  line L4271 (24.6851, -58.8002) -> (24.6851, -58.294)
  line L4272 (24.3803, -57.3016) -> (24.3803, -56.7954)
  line L4273 (24.6851, -57.3016) -> (24.3803, -57.3016)
  line L4274 (24.6851, -56.7954) -> (24.6851, -57.3016)
  line L4275 (24.3803, -56.7954) -> (24.6851, -56.7954)
  line L4276 (46.5113, -20.2852) -> (46.5113, -20.6114)
  line L4277 (46.5113, -18.7589) -> (46.5113, -19.0849)
  line L4278 (43.6589, -18.7589) -> (46.5113, -18.7589)
  line L4279 (43.6589, -20.6114) -> (46.5113, -20.6114)
  line L4280 (44.1137, -20.6112) -> (44.1137, -18.7588)
  line L4281 (43.4303, -20.1812) -> (43.4303, -20.6874)
  line L4282 (43.7351, -20.6874) -> (43.7351, -20.1812)
  line L4283 (43.7351, -20.1812) -> (43.4303, -20.1812)
  line L4284 (43.4303, -20.6874) -> (43.7351, -20.6874)
  line L4285 (43.7351, -19.1888) -> (43.4303, -19.1888)
  line L4286 (43.4303, -19.1888) -> (43.4303, -18.6826)
  line L4287 (43.7351, -18.6826) -> (43.7351, -19.1888)
  line L4288 (43.4303, -18.6826) -> (43.7351, -18.6826)
  line L4289 (46.5113, -58.3979) -> (46.5113, -58.7242)
  line L4290 (46.5113, -56.8716) -> (46.5113, -57.1977)
  line L4291 (43.6589, -56.8716) -> (46.5113, -56.8716)
  line L4292 (43.6589, -58.7242) -> (46.5113, -58.7242)
  line L4293 (44.1137, -58.724) -> (44.1137, -56.8716)
  line L4294 (43.4303, -58.8002) -> (43.7351, -58.8002)
  line L4295 (43.7351, -58.294) -> (43.4303, -58.294)
  line L4296 (43.4303, -58.294) -> (43.4303, -58.8002)
  line L4297 (43.7351, -58.8002) -> (43.7351, -58.294)
  line L4298 (43.4303, -57.3016) -> (43.4303, -56.7954)
  line L4299 (43.7351, -57.3016) -> (43.4303, -57.3016)
  line L4300 (43.7351, -56.7954) -> (43.7351, -57.3016)
  line L4301 (43.4303, -56.7954) -> (43.7351, -56.7954)
  line L4302 (46.5113, -39.3352) -> (46.5113, -39.6614)
  line L4303 (46.5113, -37.8089) -> (46.5113, -38.135)
  line L4304 (43.6589, -37.8089) -> (46.5113, -37.8089)
  line L4305 (43.6589, -39.6614) -> (46.5113, -39.6614)
  line L4306 (44.1137, -39.6613) -> (44.1137, -37.8089)
  line L4307 (43.4303, -39.7375) -> (43.7351, -39.7375)
  line L4308 (43.7351, -39.2313) -> (43.4303, -39.2313)
  line L4309 (43.7351, -39.7375) -> (43.7351, -39.2313)
  line L4310 (43.4303, -39.2313) -> (43.4303, -39.7375)
  line L4311 (43.7351, -37.7327) -> (43.7351, -38.2389)
  line L4312 (43.4303, -38.2389) -> (43.4303, -37.7327)
  line L4313 (43.4303, -37.7327) -> (43.7351, -37.7327)
  line L4314 (43.7351, -38.2389) -> (43.4303, -38.2389)
  line L4315 (217.9616, -20.2852) -> (217.9616, -20.6114)
  line L4316 (217.9616, -18.7589) -> (217.9616, -19.0849)
  line L4317 (215.1092, -18.7589) -> (217.9616, -18.7589)
  line L4318 (215.1092, -20.6114) -> (217.9616, -20.6114)
  line L4319 (215.564, -20.6112) -> (215.564, -18.7588)
  line L4320 (215.1854, -20.1812) -> (214.8806, -20.1812)
  line L4321 (214.8806, -20.6874) -> (215.1854, -20.6874)
  line L4322 (215.1854, -20.6874) -> (215.1854, -20.1812)
  line L4323 (214.8806, -20.1812) -> (214.8806, -20.6874)
  line L4324 (214.8806, -18.6826) -> (215.1854, -18.6826)
  line L4325 (215.1854, -19.1888) -> (214.8806, -19.1888)
  line L4326 (215.1854, -18.6826) -> (215.1854, -19.1888)
  line L4327 (214.8806, -19.1888) -> (214.8806, -18.6826)
  line L4328 (217.9616, -77.4607) -> (217.9616, -77.7869)
  line L4329 (217.9616, -75.9344) -> (217.9616, -76.2604)
  line L4330 (215.1092, -75.9344) -> (217.9616, -75.9344)
  line L4331 (215.1092, -77.7869) -> (217.9616, -77.7869)
  line L4332 (215.564, -77.7867) -> (215.564, -75.9343)
  line L4333 (215.1854, -77.3568) -> (214.8806, -77.3568)
  line L4334 (214.8806, -77.3568) -> (214.8806, -77.863)
  line L4335 (215.1854, -77.863) -> (215.1854, -77.3568)
  line L4336 (214.8806, -77.863) -> (215.1854, -77.863)
  line L4337 (215.1854, -76.3644) -> (214.8806, -76.3644)
  line L4338 (215.1854, -75.8582) -> (215.1854, -76.3644)
  line L4339 (214.8806, -76.3644) -> (214.8806, -75.8582)
  line L4340 (214.8806, -75.8582) -> (215.1854, -75.8582)
  line L4341 (217.9616, -58.3979) -> (217.9616, -58.7242)
  line L4342 (217.9616, -56.8716) -> (217.9616, -57.1977)
  line L4343 (215.1092, -56.8716) -> (217.9616, -56.8716)
  line L4344 (215.1092, -58.7242) -> (217.9616, -58.7242)
  line L4345 (215.564, -58.724) -> (215.564, -56.8716)
  line L4346 (214.8806, -58.294) -> (214.8806, -58.8002)
  line L4347 (215.1854, -58.294) -> (214.8806, -58.294)
  line L4348 (214.8806, -58.8002) -> (215.1854, -58.8002)
  line L4349 (215.1854, -58.8002) -> (215.1854, -58.294)
  line L4350 (215.1854, -57.3016) -> (214.8806, -57.3016)
  line L4351 (214.8806, -57.3016) -> (214.8806, -56.7954)
  line L4352 (214.8806, -56.7954) -> (215.1854, -56.7954)
  line L4353 (215.1854, -56.7954) -> (215.1854, -57.3016)
  line L4354 (217.9616, -39.3352) -> (217.9616, -39.6614)
  line L4355 (217.9616, -37.8089) -> (217.9616, -38.135)
  line L4356 (215.1092, -37.8089) -> (217.9616, -37.8089)
  line L4357 (215.1092, -39.6614) -> (217.9616, -39.6614)
  line L4358 (215.564, -39.6613) -> (215.564, -37.8089)
  line L4359 (214.8806, -39.7375) -> (215.1854, -39.7375)
  line L4360 (215.1854, -39.2313) -> (214.8806, -39.2313)
  line L4361 (214.8806, -39.2313) -> (214.8806, -39.7375)
  line L4362 (215.1854, -39.7375) -> (215.1854, -39.2313)
  line L4363 (215.1854, -37.7327) -> (215.1854, -38.2389)
  line L4364 (214.8806, -37.7327) -> (215.1854, -37.7327)
  line L4365 (215.1854, -38.2389) -> (214.8806, -38.2389)
  line L4366 (214.8806, -38.2389) -> (214.8806, -37.7327)
  line L4367 (198.9116, -39.3352) -> (198.9116, -39.6614)
  line L4368 (198.9116, -37.8089) -> (198.9116, -38.135)
  line L4369 (196.0592, -37.8089) -> (198.9116, -37.8089)
  line L4370 (196.0592, -39.6614) -> (198.9116, -39.6614)
  line L4371 (196.514, -39.6613) -> (196.514, -37.8089)
  line L4372 (196.1354, -39.7375) -> (196.1354, -39.2313)
  line L4373 (195.8306, -39.2313) -> (195.8306, -39.7375)
  line L4374 (195.8306, -39.7375) -> (196.1354, -39.7375)
  line L4375 (196.1354, -39.2313) -> (195.8306, -39.2313)
  line L4376 (196.1354, -37.7327) -> (196.1354, -38.2389)
  line L4377 (196.1354, -38.2389) -> (195.8306, -38.2389)
  line L4378 (195.8306, -38.2389) -> (195.8306, -37.7327)
  line L4379 (195.8306, -37.7327) -> (196.1354, -37.7327)
  line L4380 (198.9116, -77.4607) -> (198.9116, -77.7869)
  line L4381 (198.9116, -75.9344) -> (198.9116, -76.2604)
  line L4382 (196.0592, -75.9344) -> (198.9116, -75.9344)
  line L4383 (196.0592, -77.7869) -> (198.9116, -77.7869)
  line L4384 (196.514, -77.7867) -> (196.514, -75.9343)
  line L4385 (196.1354, -77.3568) -> (195.8306, -77.3568)
  line L4386 (195.8306, -77.863) -> (196.1354, -77.863)
  line L4387 (195.8306, -77.3568) -> (195.8306, -77.863)
  line L4388 (196.1354, -77.863) -> (196.1354, -77.3568)
  line L4389 (196.1354, -76.3644) -> (195.8306, -76.3644)
  line L4390 (195.8306, -75.8582) -> (196.1354, -75.8582)
  line L4391 (195.8306, -76.3644) -> (195.8306, -75.8582)
  line L4392 (196.1354, -75.8582) -> (196.1354, -76.3644)
  line L4393 (198.9116, -58.3979) -> (198.9116, -58.7242)
  line L4394 (198.9116, -56.8716) -> (198.9116, -57.1977)
  line L4395 (196.0592, -56.8716) -> (198.9116, -56.8716)
  line L4396 (196.0592, -58.7242) -> (198.9116, -58.7242)
  line L4397 (196.514, -58.724) -> (196.514, -56.8716)
  line L4398 (195.8306, -58.294) -> (195.8306, -58.8002)
  line L4399 (196.1354, -58.8002) -> (196.1354, -58.294)